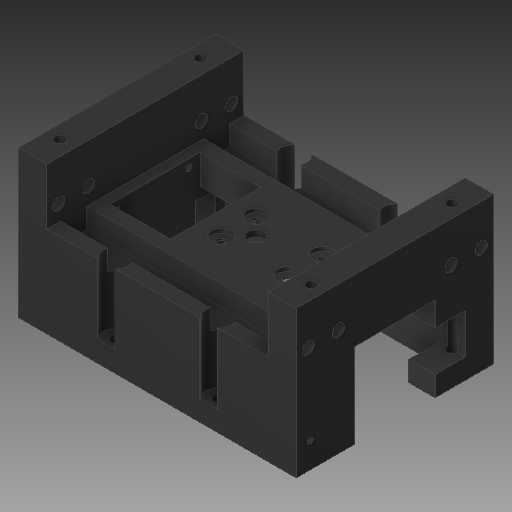
# Autodesk Inventor part: GA01
Saved by Autodesk Inventor 2017 (Build 210142000, 142)
## iProperties
Created: 2018-10-23
Part Number: GA01
Material: ABS Plastic
Document SubType Name: Modeling
Designer: Dell
Density: 1.06 g/cm^3
Appearance: Smooth - Black
Author: Dell
Autodesk Inventor part; units mm, degrees
ref_plane "YZ Plane" through (0, 0, 0) normal (1, 0, 0) x (0, 1, 0)
ref_plane "XZ Plane" through (0, 0, 0) normal (0, 1, 0) x (-1, 0, 0)
sketch "Sketch26" plane through (0, 0, 0) normal (0, 0, 1) x (1, 0, 0)
  line L0 (0, 0) -> (140, 0)
  line L1 (140, 0) -> (140, 48)
  line L2 (140, 48) -> (0, 48)
  line L3 (0, 48) -> (0, 0)
  dimension "d137" = 48
  dimension "d138" = 140
  constraints: 8 end point, 2 parallel, 1 horizontal, 1 perpendicular
  measures "d137" distance of L1.end L0.end
  measures "d138" distance of L1.end L2.end
extrude "Extrusion22" add sketch "Sketch26" along normal blind 100
sketch "Sketch27" plane through (0, 48, 0) normal (0, 1, 0) x (1, 0, 0)
  line L0 (0, -100) -> (140, -100) projected
  line L1 (0, 0) -> (140, 0) projected
  line L2 (15, -100) -> (125, -100)
  line L3 (125, -100) -> (125, 0)
  line L4 (125, 0) -> (15, 0)
  line L5 (15, 0) -> (15, -100)
  line L6 (0, 0) -> (0, -100) projected
  line L7 (140, -100) -> (0, -100) projected
  point P0 (70, -100)
  point P1 (70, -100)
  dimension "d141" = 15
  constraints: 8 end point, 4 midpoint, 2 parallel, 2 point on line, 1 horizontal, 1 perpendicular
  measures "d141" distance between parallel lines of L6 L5
extrude "Extrusion23" cut sketch "Sketch27" against normal blind 28 contours L5 L1 L3 L0
sketch "Sketch28" plane through (140, 0, 0) normal (1, 0, 0) x (0, 0, -1)
  circle A0 centre (-93, 28) radius 3
  circle A1 centre (-78, 28) radius 3
  line L0 (-93, 28) -> (-78, 28) construction
  line L1 (0, 48) -> (-100, 48) construction
  line L2 (-50, 48) -> (-50, 0) construction
  line L3 (0, 0) -> (-100, 0) construction
  line L4 (-100, 48) -> (0, 48) construction
  line L5 (-100, 20) -> (-100, 48) construction
  line L6 (-100, 20) -> (0, 20) construction
  line L7 (0, 48) -> (0, 20) construction
  circle A2 centre (-7, 28) radius 3
  circle A3 centre (-22, 28) radius 3
  dimension "d144" = 6
  dimension "d145" = 6
  dimension "d146" = 15
  dimension "d173" = 28
  dimension "d177" = 8
  constraints: 4 centre point, 4 end point, 2 midpoint, 2 symmetric about line, 1 horizontal, 2 other
  measures "d144" diameter of A0
  measures "d145" diameter of A1
  measures "d146" distance of L0.start L0.end
  measures "d173" distance from line of L2 L0.end
  measures "d177" distance from line of L6 L0.start
extrude "Extrusion24" cut sketch "Sketch28" against normal through all
sketch "Sketch30" plane through (0, 0, 0) normal (0, -1, 0) x (1, 0, 0)
  line L0 (63.5, 63.5) -> (39.5, 63.5) construction
  line L1 (39.5, 63.5) -> (39.5, 36.5) construction
  line L2 (39.5, 36.5) -> (63.5, 36.5) construction
  line L3 (63.5, 36.5) -> (63.5, 63.5) construction
  circle A0 centre (70, 50) radius 12.5
  line L4 (140, 0) -> (140, 100) projected
  line L5 (0, 100) -> (140, 100) projected
  circle A1 centre (63.5, 63.5) radius 1.5
  circle A2 centre (63.5, 36.5) radius 1.5
  circle A3 centre (55.5, 63.5) radius 1.5
  circle A4 centre (55.5, 36.5) radius 1.5
  circle A5 centre (47.5, 63.5) radius 1.5
  circle A6 centre (47.5, 36.5) radius 1.5
  circle A7 centre (39.5, 63.5) radius 1.5
  circle A8 centre (39.5, 36.5) radius 1.5
  point P0 (0, 0)
  point P1 (63.5, 50)
  point P2 (140, 50)
  point P3 (70, 100)
  dimension "d153" = 24
  dimension "d154" = 27
  dimension "d155" = 6.5
  dimension "d156" = 25
  dimension "d157" = 3
  dimension "d158" = 3
  dimension "d161" = 8
  constraints: 9 centre point, 8 end point, 3 midpoint, 2 coincident, 2 horizontal, 2 horizontal alignment, 2 parallel, 1 perpendicular, 1 vertical alignment, 12 other
  measures "d153" distance of L2.end L1.end
  measures "d154" distance of L1.end L0.end
  measures "d155" distance from line of L3 A0.centre
  measures "d156" diameter of A0
  measures "d157" diameter of A1
  measures "d158" diameter of A2
  measures "d161" distance of A1.centre A3.centre
extrude "Extrusion26" cut sketch "Sketch30" against normal through all
sketch "Sketch31" plane through (0, 0, 0) normal (0, -1, 0) x (1, 0, 0)
  line L0 (84, 70) -> (29, 70)
  line L1 (29, 70) -> (29, 30)
  line L2 (29, 30) -> (84, 30)
  line L3 (84, 30) -> (84, 70)
  circle A0 centre (70, 50) radius 12.5 projected
  point P0 (0, 0)
  point P1 (84, 50)
  dimension "d168" = 55
  dimension "d169" = 40
  dimension "d170" = 14
  constraints: 8 end point, 2 parallel, 1 horizontal, 1 horizontal alignment, 1 midpoint, 1 perpendicular
  measures "d168" distance of L1.end L2.end
  measures "d169" distance of L2.end L0.start
  measures "d170" distance from line of L3 A0.centre
extrude "Extrusion27" cut sketch "Sketch31" against normal blind 17 contours L3 L2 L1 L0 | A0
sketch "Sketch32" plane through (0, 0, 0) normal (0, -1, 0) x (1, 0, 0)
  line L0 (84, 30) -> (29, 30) projected
  line L1 (29, 30) -> (29, 70) projected
  line L2 (29, 70) -> (84, 70) projected
  line L3 (84, 70) -> (84, 30) projected
  line L4 (84, 30) -> (29, 30) projected
  line L5 (0, 0) -> (140, 0) projected
  line L6 (140, 0) -> (140, 100) projected
  line L7 (0, 100) -> (140, 100) projected
  line L8 (0, 0) -> (0, 100) projected
extrude "Extrusion28" add sketch "Sketch32" along normal blind 25
sketch "Sketch33" plane through (0, 20, 0) normal (0, 1, 0) x (1, 0, 0)
  circle A0 centre (70, -50) radius 12.5 construction
  line L0 (44.5, -94.1673) -> (19, -50) construction
  line L1 (19, -50) -> (44.5, -5.8327) construction
  line L2 (44.5, -5.8327) -> (95.5, -5.8327) construction
  line L3 (95.5, -5.8327) -> (121, -50) construction
  line L4 (121, -50) -> (95.5, -94.1673) construction
  line L5 (95.5, -94.1673) -> (44.5, -94.1673) construction
  circle A1 centre (121, -50) radius 2.5
  circle A2 centre (95.5, -94.1673) radius 2.5
  circle A3 centre (44.5, -94.1673) radius 2.5
  circle A4 centre (19, -50) radius 2.5
  circle A5 centre (44.5, -5.8327) radius 2.5
  circle A6 centre (95.5, -5.8327) radius 2.5
  point P0 (0, 0)
  point P1 (70, -50)
  dimension "d178" = 102
  dimension "d179" = 5
  dimension "d180" = 5
  dimension "d181" = 5
  dimension "d182" = 5
  dimension "d183" = 5
  dimension "d184" = 5
  constraints: 12 end point, 7 coincident, 6 centre point, 1 horizontal, 13 other
  measures "d178" distance of L0.end L3.end
  measures "d179" diameter of A1
  measures "d180" diameter of A2
  measures "d181" diameter of A3
  measures "d182" diameter of A4
  measures "d183" diameter of A5
  measures "d184" diameter of A6
extrude "Extrusion29" cut sketch "Sketch33" against normal through all
sketch "Sketch34" plane through (0, 20, 0) normal (0, 1, 0) x (1, 0, 0)
  circle A0 centre (70, -50) radius 12.5 projected
  circle A1 centre (95.5, -5.8327) radius 2.5 projected
  circle A2 centre (95.5, -5.8327) radius 6.5
  circle A3 centre (44.5, -5.8327) radius 6.5
  circle A4 centre (19, -50) radius 6.5
  circle A5 centre (44.5, -94.1673) radius 6.5
  circle A6 centre (95.5, -94.1673) radius 6.5
  circle A7 centre (121, -50) radius 6.5
  point P0 (0, 0)
  dimension "d187" = 13
  dimension "d190" = 360
  constraints: 6 centre point, 1 coincident, 13 other
  measures "d187" diameter of A2
extrude "Extrusion30" cut sketch "Sketch34" along normal blind 50 and the other way blind 35 contours A0 | A1 | A2 | A3 | A4 | A5 | A6 | A7
sketch "Sketch35" plane through (0, -25, 0) normal (0, -1, 0) x (1, 0, 0)
  circle A0 centre (44.5, 5.8327) radius 2.5 construction
  circle A1 centre (44.5, 94.1673) radius 2.5 construction
  circle A2 centre (121, 50) radius 2.5 construction
  circle A3 centre (95.5, 94.1673) radius 2.5 construction
  circle A4 centre (19, 50) radius 2.5 construction
  circle A5 centre (95.5, 5.8327) radius 2.5 construction
  line L0 (29, 70) -> (84, 70) projected
  line L1 (84, 70) -> (84, 30) projected
  line L2 (84, 30) -> (29, 30) projected
  line L3 (29, 30) -> (29, 70) projected
  line L4 (0, 0) -> (140, 0) construction
  line L5 (140, 0) -> (140, 100) construction
  line L6 (140, 100) -> (0, 100) construction
  line L7 (0, 100) -> (0, 0) construction
  line L8 (84, 30) -> (111, 30)
  line L9 (111, 30) -> (111, 70)
  line L10 (111, 70) -> (84, 70)
  line L11 (84, 70) -> (84, 30)
  dimension "d196" = 27
  constraints: 8 end point, 2 parallel, 1 horizontal, 1 horizontal alignment, 1 perpendicular
  measures "d196" distance of L1.end L8.end
extrude "Extrusion31" cut sketch "Sketch35" against normal blind 25 contours L10 L9 L8 L1
sketch "Sketch36" plane through (140, 48, 100) normal (0, 1, 0) x (1, 0, 0)
  line L0 (-7.5, 15) -> (-7.5, 85) construction
  circle A0 centre (-7.5, 15) radius 2.5
  circle A1 centre (-7.5, 85) radius 2.5
  line L1 (0, 0) -> (-15, 0) construction
  line L2 (0, 100) -> (0, 0) construction
  circle A2 centre (-70, 50) radius 12.5 construction
  line L3 (-70, 50) -> (-70, 0) construction
  line L4 (-47.3687, 0) -> (-92.6313, 0) construction
  circle A3 centre (-132.5, 15) radius 2.5
  circle A4 centre (-132.5, 85) radius 2.5
  point P0 (-7.5, 50)
  point P1 (-7.5, 0)
  point P2 (0, 50)
  dimension "d199" = 5
  dimension "d200" = 5
  dimension "d201" = 70
  constraints: 4 centre point, 4 end point, 4 midpoint, 2 coincident, 2 symmetric about line, 2 vertical, 1 horizontal alignment, 1 vertical alignment, 2 other
  measures "d199" diameter of A0
  measures "d200" diameter of A1
  measures "d201" distance of L0.start L0.end
extrude "Extrusion32" cut sketch "Sketch36" against normal through all
sketch "Sketch37" plane through (0, 0, 0) normal (0, -1, 0) x (1, 0, 0)
  line L0 (84, 62.0836) -> (140, 62.0836)
  line L1 (140, 62.0836) -> (140, 82.0836)
  line L2 (140, 82.0836) -> (84, 82.0836)
  line L3 (84, 82.0836) -> (84, 62.0836)
  arc A0 (92.6313, 100) -> (98.3687, 100) centre (95.5, 94.1673) ccw construction
  arc A1 (125, 55.1235) -> (125, 44.8765) centre (121, 50) ccw construction
  line L4 (95.5, 94.1673) -> (121, 94.1673) construction
  line L5 (121, 94.1673) -> (121, 50) construction
  line L6 (84, 70) -> (84, 30) projected
  line L7 (140, 0) -> (140, 100) projected
  point P0 (0, 0)
  point P1 (84, 72.0836)
  point P2 (121, 72.0836)
  dimension "d204" = 20
  constraints: 12 end point, 2 horizontal, 2 midpoint, 2 parallel, 2 perpendicular, 2 point on line, 1 horizontal alignment
  measures "d204" distance of L0.end L1.end
extrude "Extrusion33" cut sketch "Sketch37" along normal blind 20
sketch "Sketch38" plane through (0, 48, 100) normal (0, 1, 0) x (1, 0, 0)
  line L0 (15, 0) -> (0, 0) projected
  line L1 (140, 100) -> (125, 100) projected
  line L2 (0, 100) -> (0, 0) projected
  line L3 (140, 100) -> (140, 0) projected
  line L4 (0, 0) -> (140, 0)
  line L5 (140, 0) -> (140, 100)
  line L6 (140, 100) -> (0, 100)
  line L7 (0, 100) -> (0, 0)
  line L8 (139, 1) -> (1, 1)
  line L9 (1, 1) -> (1, 99)
  line L10 (1, 99) -> (139, 99)
  line L11 (139, 99) -> (139, 1)
  dimension "d207" = 1
  constraints: 16 end point, 4 parallel, 2 perpendicular, 1 horizontal, 3 other
  measures "d207" distance between parallel lines of L4 L8
extrude "Extrusion34" cut sketch "Sketch38" against normal through all
sketch "Sketch39" plane through (0, 0, 0) normal (0, -1, 0) x (1, 0, 0)
  line L0 (139, 62.0836) -> (139, 82.0836) projected
  line L1 (139, 82.0836) -> (84, 82.0836) projected
  line L2 (84, 82.0836) -> (84, 70) projected
  line L3 (84, 30) -> (84, 70) projected
  line L4 (111, 30) -> (84, 30) projected
  line L5 (111, 62.0836) -> (111, 30) projected
  line L6 (111, 62.0836) -> (139, 62.0836) projected
  arc A0 (48.8468, 1) -> (40.1532, 1) centre (44.5, 5.8327) ccw projected
  arc A1 (99.8468, 1) -> (91.1532, 1) centre (95.5, 5.8327) ccw projected
  arc A2 (40.1532, 99) -> (48.8468, 99) centre (44.5, 94.1673) ccw projected
  circle A3 centre (19, 50) radius 6.5 projected
  arc A4 (91.1532, 99) -> (99.8468, 99) centre (95.5, 94.1673) ccw projected
  circle A5 centre (121, 50) radius 6.5 projected
  line L7 (127.5, 82.0836) -> (19, 82.0836)
  line L8 (19, 82.0836) -> (19, 86.1673)
  line L9 (19, 86.1673) -> (127.5, 86.1673)
  line L10 (127.5, 86.1673) -> (127.5, 82.0836)
  line L11 (29, 70) -> (84, 70) projected
  line L12 (84, 70) -> (19, 70)
  line L13 (19, 70) -> (19, 82.0836)
  line L14 (19, 82.0836) -> (84, 82.0836)
  line L15 (84, 82.0836) -> (84, 70)
  line L16 (111, 42) -> (127.5, 42)
  line L17 (127.5, 42) -> (127.5, 13.8327)
  line L18 (127.5, 13.8327) -> (111, 13.8327)
  line L19 (111, 13.8327) -> (111, 42)
  line L20 (127.5, 13.8327) -> (19, 13.8327)
  line L21 (19, 13.8327) -> (19, 30)
  line L22 (19, 30) -> (127.5, 30)
  line L23 (127.5, 30) -> (127.5, 13.8327)
  circle A6 centre (132.5, 85) radius 2.5 projected
  point P0 (0, 0)
  point P1 (29, 30)
  dimension "d210" = 5
  dimension "d211" = 8
  dimension "d212" = 8
  dimension "d213" = 8
  constraints: 32 end point, 8 parallel, 4 horizontal, 4 perpendicular, 3 point on line, 3 vertical alignment
  measures "d210" distance from line of L10 A6.centre
  measures "d211" distance from line of A0.centre L20
  measures "d212" distance from line of L16 A5.centre
  measures "d213" distance from line of A2.centre L9
extrude "Extrusion35" cut sketch "Sketch39" along normal through all contours L6 L5 L4 L3 L2 L1 L0 | L1 L7 L8 L9 L10 | L2 L11 L12 L13 L7 | L19 L20 L21 L22 L4 | L22 L17 L18 L19
sketch "Sketch41" plane through (1, 48, 1) normal (-1, 0, 0) x (0, 0, 1)
  line L0 (69, -48) -> (69, -73) projected
  line L1 (69, -48) -> (69, -73) projected
  line L2 (29, -73) -> (29, -48) projected
  line L3 (29, -48) -> (29, -73) projected
  line L4 (29, -73) -> (29, -48) projected
  line L5 (29, -48) -> (69, -48)
  line L6 (69, -48) -> (69, -73)
  line L7 (69, -73) -> (29, -73)
  line L8 (29, -73) -> (29, -48)
  line L9 (29, -48) -> (19, -48)
  line L10 (19, -48) -> (19, -73)
  line L11 (19, -73) -> (29, -73)
  line L12 (29, -73) -> (29, -48)
  point P0 (-1, -48)
  dimension "d218" = 10
  constraints: 16 end point, 4 parallel, 2 horizontal, 2 perpendicular, 1 horizontal alignment
  measures "d218" distance between parallel lines of L10 L2
extrude "Extrusion36" cut sketch "Sketch41" against normal blind 5 contours L0 L7 L2 L5
extrude "Extrusion37" cut sketch "Sketch41" against normal blind 20 contours L2 L11 L10 L9
sketch "Sketch42" plane through (0, 0, 0) normal (0, -1, 0) x (1, 0, 0)
  line L0 (29, 70) -> (84, 70) projected
  line L1 (19, 86.1673) -> (19, 70) projected
  line L2 (29, 70) -> (19, 70)
  line L3 (19, 70) -> (19, 86.1673)
  line L4 (19, 86.1673) -> (29, 86.1673)
  line L5 (29, 86.1673) -> (29, 70)
  point P0 (0, 0)
  constraints: 8 end point, 2 parallel, 1 horizontal, 1 perpendicular
extrude "Extrusion38" add sketch "Sketch42" along normal blind 25
sketch "Sketch43" plane through (0, 0, 0) normal (0, -1, 0) x (1, 0, 0)
  line L0 (111, 62.0836) -> (111, 30) projected
  line L1 (127.5, 13.8327) -> (19, 13.8327) projected
  line L2 (111, 30) -> (127.5, 30)
  line L3 (127.5, 30) -> (127.5, 13.8327)
  line L4 (127.5, 13.8327) -> (111, 13.8327)
  line L5 (111, 13.8327) -> (111, 30)
  point P0 (0, 0)
  constraints: 8 end point, 2 parallel, 1 horizontal, 1 perpendicular
extrude "Extrusion39" add sketch "Sketch43" along normal blind 25
sketch "Sketch44" plane through (0, 0, 0) normal (0, -1, 0) x (1, 0, 0)
  line L0 (139, 62.0836) -> (111, 62.0836) projected
  line L1 (111, 62.0836) -> (111, 13.8327) projected
  line L2 (139, 62.0836) -> (111, 62.0836)
  line L3 (111, 62.0836) -> (111, 57.0836)
  line L4 (111, 57.0836) -> (139, 57.0836)
  line L5 (139, 57.0836) -> (139, 62.0836)
  point P0 (0, 0)
  dimension "d225" = 5
  constraints: 8 end point, 2 parallel, 1 horizontal, 1 perpendicular, 1 point on line
  measures "d225" distance between parallel lines of L4 L0
extrude "Extrusion40" cut sketch "Sketch44" along normal through all
sketch "Sketch45" plane through (0, 0, 0) normal (0, -1, 0) x (1, 0, 0)
  line L0 (127.5, 82.0836) -> (139, 82.0836) projected
  line L1 (139, 82.0836) -> (139, 57.0836) projected
  line L2 (127.5, 82.0836) -> (139, 82.0836)
  line L3 (139, 82.0836) -> (139, 77.0836)
  line L4 (139, 77.0836) -> (127.5, 77.0836)
  line L5 (127.5, 77.0836) -> (127.5, 82.0836)
  point P0 (0, 0)
  dimension "d228" = 5
  constraints: 8 end point, 2 parallel, 1 horizontal, 1 perpendicular, 1 point on line
  measures "d228" distance between parallel lines of L0 L4
extrude "Extrusion41" add sketch "Sketch45" along normal blind 25
sketch "Sketch46" plane through (0, 0, 0) normal (0, -1, 0) x (1, 0, 0)
  line L0 (127.5, 77.0836) -> (139, 77.0836) projected
  line L1 (29, 86.1673) -> (127.5, 86.1673) projected
  line L2 (127.5, 77.0836) -> (29, 77.0836)
  line L3 (29, 77.0836) -> (29, 86.1673)
  line L4 (29, 86.1673) -> (127.5, 86.1673)
  line L5 (127.5, 86.1673) -> (127.5, 77.0836)
  point P0 (0, 0)
  constraints: 8 end point, 2 parallel, 1 horizontal, 1 perpendicular
extrude "Extrusion42" add sketch "Sketch46" along normal blind 25
sketch "Sketch47" plane through (0, 0, 0) normal (0, -1, 0) x (1, 0, 0)
  line L0 (29, 30) -> (29, 70) projected
  line L1 (29, 77.0836) -> (139, 77.0836) projected
  line L2 (29, 70) -> (84, 70)
  line L3 (84, 70) -> (84, 77.0836)
  line L4 (84, 77.0836) -> (29, 77.0836)
  line L5 (29, 77.0836) -> (29, 70)
  point P0 (0, 0)
  constraints: 8 end point, 2 parallel, 1 horizontal, 1 midpoint, 1 perpendicular
extrude "Extrusion43" add sketch "Sketch47" along normal blind 25
sketch "Sketch48" plane through (0, 0, 0) normal (0, -1, 0) x (1, 0, 0)
  line L0 (84, 77.0836) -> (84, 70) construction
  line L1 (84, 30) -> (84, 70) construction
  line L2 (29, 30) -> (84, 30) construction
  line L3 (29, 30) -> (6, 30) construction
  line L4 (6, 30) -> (6, 70) construction
  line L5 (1, 70) -> (6, 70) construction
  line L6 (1, 20) -> (1, 70) construction
  line L7 (1, 20) -> (19, 20) construction
  line L8 (19, 20) -> (19, 13.8327) construction
  line L9 (19, 13.8327) -> (111, 13.8327) construction
  line L10 (111, 13.8327) -> (111, 57.0836) construction
  line L11 (111, 57.0836) -> (139, 57.0836) construction
  line L12 (139, 77.0836) -> (139, 57.0836) construction
  line L13 (139, 77.0836) -> (84, 77.0836) construction
  circle A0 centre (97.5, 25.4582) radius 1.5
  circle A1 centre (97.5, 40.4582) radius 1.5
  line L14 (111, 57.0836) -> (84, 57.0836) construction
  line L15 (84, 70) -> (84, 30) construction
  line L16 (97.5, 25.4582) -> (97.5, 40.4582) construction
  point P0 (0, 0)
  point P1 (97.5, 57.0836)
  point P2 (97.5, 32.9582)
  point P3 (111, 35.4582)
  dimension "d235" = 3
  dimension "d236" = 3
  dimension "d276" = 11.6255
  dimension "d277" = 15
  constraints: 4 end point, 3 midpoint, 2 centre point, 1 perpendicular, 1 point on line, 1 vertical, 1 vertical alignment
  measures "d235" diameter of A0
  measures "d236" diameter of A1
  measures "d276" distance from line of L9 L16.start
  measures "d277" distance of L16.start L16.end
extrude "Extrusion44" cut sketch "Sketch48" against normal blind 12
sketch "Sketch49" plane through (6, 48, 1) normal (-1, 0, 0) x (0, 0, 1)
  line L0 (69, -48) -> (69, -73) projected
  line L1 (29, -48) -> (69, -48) projected
  line L2 (29, -73) -> (29, -48) projected
  line L3 (69, -73) -> (29, -73) projected
  circle A0 centre (34, -68) radius 1.5
  circle A1 centre (64, -68) radius 1.5
  point P0 (-1, -48)
  dimension "d240" = 3
  dimension "d241" = 3
  dimension "d244" = 5
  dimension "d245" = 5
  dimension "d260" = 5
  constraints: 2 centre point, 1 horizontal alignment
  measures "d240" diameter of A0
  measures "d241" diameter of A1
  measures "d244" distance from line of L0 A1.centre
  measures "d245" distance from line of L3 A1.centre
  measures "d260" distance from line of L2 A0.centre
extrude "Extrusion45" cut sketch "Sketch49" against normal blind 25 contours A0 | A1
sketch "Sketch50" plane through (1, 48, 1) normal (-1, 0, 0) x (0, 0, 1)
  circle A0 centre (91, -60.5) radius 1.5
  circle A1 centre (7, -60.5) radius 1.5
  line L0 (69, -48) -> (69, -73) projected
  line L1 (0, 0) -> (0, -73) projected
  line L2 (98, 0) -> (98, -73) projected
  point P0 (-1, -48)
  point P1 (69, -60.5)
  point P2 (69, -60.5)
  dimension "d248" = 3
  dimension "d249" = 3
  dimension "d250" = 7
  dimension "d251" = 7
  constraints: 2 centre point, 2 horizontal alignment, 2 midpoint
  measures "d248" diameter of A0
  measures "d249" diameter of A1
  measures "d250" distance from line of L1 A1.centre
  measures "d251" distance from line of L2 A0.centre
extrude "Extrusion46" cut sketch "Sketch50" against normal blind 12
sketch "Sketch52" plane through (0, 0, 0) normal (0, -1, 0) x (1, 0, 0)
  circle A0 centre (97.5, 25.4582) radius 1.5 projected
  circle A1 centre (97.5, 40.4582) radius 1.5 projected
  line L0 (84, 77.0836) -> (84, 70) projected
  line L1 (84, 30) -> (84, 70) projected
  line L2 (29, 30) -> (84, 30) projected
  line L3 (29, 30) -> (6, 30) projected
  line L4 (6, 30) -> (6, 70) projected
  line L5 (1, 70) -> (6, 70) projected
  line L6 (1, 20) -> (1, 70) projected
  line L7 (1, 20) -> (19, 20) projected
  line L8 (19, 20) -> (19, 13.8327) projected
  line L9 (19, 13.8327) -> (111, 13.8327) projected
  line L10 (111, 13.8327) -> (111, 57.0836) projected
  line L11 (111, 57.0836) -> (139, 57.0836) projected
  line L12 (139, 77.0836) -> (139, 57.0836) projected
  line L13 (139, 77.0836) -> (84, 77.0836) projected
  line L14 (138, 58.0836) -> (85, 58.0836)
  line L15 (85, 58.0836) -> (85, 76.0836)
  line L16 (85, 76.0836) -> (138, 76.0836)
  line L17 (138, 76.0836) -> (138, 58.0836)
  line L18 (85, 76.0836) -> (110, 76.0836)
  line L19 (110, 76.0836) -> (110, 15.0836)
  line L20 (110, 15.0836) -> (85, 15.0836)
  line L21 (85, 15.0836) -> (85, 76.0836)
  point P0 (0, 0)
  dimension "d254" = 18
  dimension "d255" = 53
  dimension "d256" = 43
  dimension "d257" = 25
  dimension "d258" = 1
  dimension "d259" = 1
  constraints: 16 end point, 4 parallel, 2 horizontal, 2 perpendicular
  measures "d254" distance of L16.end L14.start
  measures "d255" distance of L15.end L16.end
  measures "d256" distance between parallel lines of L14 L20
  measures "d257" distance of L19.end L20.end
  measures "d258" distance from line of L0.end L21
  measures "d259" distance between parallel lines of L13 L16
sketch "Sketch54" plane through (0, 17, 0) normal (0, -1, 0) x (1, 0, 0)
  circle A0 centre (70, 50) radius 12.5 construction
  line L0 (36.7, 60) -> (61.2, 60) construction
  line L1 (61.2, 60) -> (61.2, 40)
  line L2 (61.2, 40) -> (36.7, 40)
  line L3 (36.7, 40) -> (36.7, 60)
  line L4 (62.2, 61) -> (35.7, 61)
  line L5 (35.7, 61) -> (35.7, 39)
  line L6 (35.7, 39) -> (62.2, 39)
  line L7 (62.2, 39) -> (62.2, 61)
  point P0 (61.2, 50)
  dimension "d278" = 8.8
  dimension "d279" = 20
  dimension "d280" = 24.5
  dimension "d281" = 1
  constraints: 16 end point, 4 parallel, 2 perpendicular, 1 horizontal, 1 horizontal alignment, 1 midpoint, 3 other
  measures "d278" distance from line of A0.centre L1
  measures "d279" distance of L2.end L0.start
  measures "d280" distance of L0.start L0.end
  measures "d281" distance between parallel lines of L0 L4
extrude "Extrusion47" cut sketch "Sketch54" against normal through all
sketch "Sketch55" plane through (0, 20, 0) normal (0, 1, 0) x (1, 0, 0)
  circle A0 centre (39.5, -36.5) radius 1.5 projected
  circle A1 centre (47.5, -36.5) radius 1.5 projected
  circle A2 centre (55.5, -36.5) radius 1.5 projected
  circle A3 centre (63.5, -36.5) radius 1.5 projected
  circle A4 centre (63.5, -63.5) radius 1.5 projected
  circle A5 centre (55.5, -63.5) radius 1.5 projected
  circle A6 centre (47.5, -63.5) radius 1.5 projected
  circle A7 centre (39.5, -63.5) radius 1.5 projected
  circle A8 centre (39.5, -36.5) radius 1.5 projected
  circle A9 centre (39.5, -36.5) radius 2.5
  circle A10 centre (47.5, -36.5) radius 1.5 projected
  circle A11 centre (47.5, -36.5) radius 2.5
  circle A12 centre (55.5, -36.5) radius 2.5
  circle A13 centre (63.5, -36.5) radius 2.5
  circle A14 centre (63.5, -63.5) radius 2.5
  circle A15 centre (55.5, -63.5) radius 1.5 projected
  circle A16 centre (55.5, -63.5) radius 2.5
  circle A17 centre (47.5, -63.5) radius 1.5 projected
  circle A18 centre (47.5, -63.5) radius 2.5
  circle A19 centre (39.5, -63.5) radius 2.5
  point P0 (0, 0)
  dimension "d284" = 5
  dimension "d285" = 5
  dimension "d286" = 5
  dimension "d287" = 5
  dimension "d288" = 5
  dimension "d289" = 5
  dimension "d290" = 5
  dimension "d291" = 5
  constraints: 8 centre point, 8 coincident
  measures "d284" diameter of A9
  measures "d285" diameter of A11
  measures "d286" diameter of A12
  measures "d287" diameter of A13
  measures "d288" diameter of A19
  measures "d289" diameter of A18
  measures "d290" diameter of A16
  measures "d291" diameter of A14
extrude "Extrusion48" cut sketch "Sketch55" against normal blind 2 contours A0 | A1 | A2 | A3 | A4 | A5 | A6 | A7 | A9 | A11 | A12 | A13 | A14 | A16 | A18 | A19
fillet "Fillet3" radius 2 2 edges at (62.2, 18.5, 59.7678) (62.2, 18.5, 40.2322)
sketch "Sketch56" plane through (0, 20, 0) normal (0, 1, 0) x (1, 0, 0)
  line L0 (1, -4) -> (1, -10)
  line L1 (15, -4) -> (15, -10)
  line L2 (1, -19) -> (1, -25)
  line L3 (15, -19) -> (15, -25)
  line L4 (125, -10) -> (125, -4)
  line L5 (15, -75) -> (15, -81)
  line L6 (15, -90) -> (15, -96)
  line L7 (15, -81) -> (15, -90)
  line L8 (15, -85.5) -> (125, -85.5)
  line L9 (15, -10) -> (15, -19)
  line L10 (15, -14.5) -> (125, -14.5)
  line L11 (15, -8) -> (125, -8)
  line L12 (125, -8) -> (125, -21)
  line L13 (125, -21) -> (15, -21)
  line L14 (15, -21) -> (15, -8)
  line L15 (15, -79) -> (125, -79)
  line L16 (125, -79) -> (125, -92)
  line L17 (125, -92) -> (15, -92)
  line L18 (15, -92) -> (15, -79)
  point P0 (0, 0)
  dimension "d295" = 13
  dimension "d296" = 13
  constraints: 38 end point, 6 midpoint, 4 parallel, 4 perpendicular, 4 point on line, 3 horizontal, 1 vertical
  measures "d295" distance between parallel lines of L13 L11
  measures "d296" distance between parallel lines of L17 L15
extrude "Extrusion49" cut sketch "Sketch56" against normal blind 10
sketch "Sketch57" plane through (0, 17, 0) normal (0, -1, 0) x (1, 0, 0)
  line L0 (29, 70) -> (84, 70) projected
  line L1 (84, 70) -> (139, 70)
  line L2 (139, 70) -> (139, 30)
  line L3 (139, 30) -> (84, 30)
  line L4 (84, 30) -> (84, 70)
  line L5 (29, 30) -> (84, 30) projected
  point P0 (0, 0)
  dimension "d299" = 55
  constraints: 8 end point, 3 point on line, 2 parallel, 1 horizontal, 1 perpendicular
  measures "d299" distance between parallel lines of L4 L2
extrude "Extrusion50" cut sketch "Sketch57" along normal through all
sketch "Sketch58" plane through (0, 17, 0) normal (0, -1, 0) x (1, 0, 0)
  arc A0 (64.0787, 38.9914) -> (64.0787, 61.0086) centre (70, 50) ccw projected
  line L0 (35.7, 61) -> (62.2, 61) projected
  circle A1 centre (121, 50) radius 6.5 projected
  arc A2 (62.2, 61) -> (64.0787, 61.0086) centre (63.1313, 62.7699) ccw projected
  arc A3 (64.0787, 38.9914) -> (64.0787, 61.0086) centre (70, 50) ccw projected
  arc A4 (64.0787, 38.9914) -> (62.2, 39) centre (63.1313, 37.2301) ccw projected
  line L1 (62.2, 39) -> (35.7, 39) projected
  line L2 (35.7, 39) -> (35.7, 61) projected
  line L3 (35.7, 61) -> (62.2, 61) projected
  line L4 (139, 70) -> (29, 70) construction
  line L5 (29, 30) -> (29, 70) projected
  line L6 (139, 30) -> (29, 30) projected
  circle A5 centre (39.5, 63.5) radius 1.5 projected
  circle A6 centre (47.5, 63.5) radius 1.5 projected
  circle A7 centre (55.5, 63.5) radius 1.5 projected
  circle A8 centre (63.5, 63.5) radius 1.5 projected
  circle A9 centre (63.5, 36.5) radius 1.5 projected
  circle A10 centre (55.5, 36.5) radius 1.5 projected
  circle A11 centre (47.5, 36.5) radius 1.5 projected
  circle A12 centre (39.5, 36.5) radius 1.5 projected
  circle A13 centre (70, 50) radius 4
  line L7 (139, 70) -> (139, 30) projected
  point P0 (0, 0)
  dimension "d302" = 8
  constraints: 1 centre point, 1 coincident
  measures "d302" diameter of A13
extrude "Extrusion51" add sketch "Sketch58" against normal blind 3 contours A4 L1 L2 L0 A2 A0 | A5 | A6 | A7 | A8 | A9 | A10 | A11 | A12
sketch "Sketch60" plane through (0, 20, 0) normal (0, 1, 0) x (1, 0, 0)
  arc A0 (64.8157, -38.6258) -> (64.3413, -38.8542) centre (63.5, -36.5) ccw projected
  circle A1 centre (55.5, -36.5) radius 2.5 projected
  circle A2 centre (47.5, -36.5) radius 1.5 projected
  circle A3 centre (47.5, -36.5) radius 2.5 projected
  circle A4 centre (39.5, -36.5) radius 2.5 projected
  circle A5 centre (39.5, -63.5) radius 2.5 projected
  circle A6 centre (47.5, -63.5) radius 2.5 projected
  circle A7 centre (55.5, -63.5) radius 2.5 projected
  arc A8 (64.3413, -61.1458) -> (64.8157, -61.3742) centre (63.5, -63.5) ccw projected
  arc A9 (64.8157, -38.6258) -> (64.3413, -38.8542) centre (70, -50) ccw projected
  arc A10 (64.8157, -38.6258) -> (64.3413, -38.8542) centre (63.5, -36.5) ccw projected
  circle A11 centre (63.5, -36.5) radius 1.5 projected
  arc A12 (64.3413, -61.1458) -> (64.8157, -61.3742) centre (70, -50) ccw projected
  arc A13 (64.3413, -61.1458) -> (64.8157, -61.3742) centre (63.5, -63.5) ccw projected
  circle A14 centre (63.5, -63.5) radius 1.5 projected
  point P0 (0, 0)
extrude "Extrusion52" add sketch "Sketch60" against normal blind 3 contours A9 A0 | A1 | A2 | A3 | A4 | A5 | A6 | A7 | A12 A8 | A11 | A14
sketch "Sketch61" plane through (0, 17, 0) normal (0, -1, 0) x (1, 0, 0)
  circle A0 centre (70, 50) radius 4 projected
  line L0 (94.5, 58.75) -> (61.5, 58.75) construction
  line L1 (61.5, 58.75) -> (61.5, 41.25) construction
  line L2 (61.5, 41.25) -> (94.5, 41.25) construction
  line L3 (94.5, 41.25) -> (94.5, 58.75) construction
  circle A1 centre (94.5, 58.75) radius 2
  circle A2 centre (61.5, 58.75) radius 2
  circle A3 centre (61.5, 41.25) radius 2
  circle A4 centre (94.5, 41.25) radius 2
  point P0 (0, 0)
  point P1 (94.5, 50)
  dimension "d307" = 33
  dimension "d308" = 17.5
  dimension "d309" = 8.5
  dimension "d310" = 4
  dimension "d311" = 4
  dimension "d312" = 4
  dimension "d313" = 4
  constraints: 8 end point, 4 centre point, 4 coincident, 2 parallel, 1 horizontal, 1 horizontal alignment, 1 midpoint, 1 perpendicular
  measures "d307" distance of L1.end L2.end
  measures "d308" distance of L2.end L0.start
  measures "d309" distance from line of L1 A0.centre
  measures "d310" diameter of A1
  measures "d311" diameter of A2
  measures "d312" diameter of A3
  measures "d313" diameter of A4
extrude "Extrusion53" cut sketch "Sketch61" against normal through all contours A1 | A2 | A3 | A4
sketch "Sketch62" plane through (0, 20, 0) normal (0, 1, 0) x (1, 0, 0)
  circle A0 centre (94.5, -41.25) radius 2 projected
  circle A1 centre (94.5, -58.75) radius 2 projected
  circle A2 centre (61.5, -58.75) radius 2 projected
  circle A3 centre (61.5, -41.25) radius 2 projected
  circle A4 centre (94.5, -41.25) radius 2 projected
  circle A5 centre (94.5, -41.25) radius 5
  circle A6 centre (94.5, -58.75) radius 5
  circle A7 centre (61.5, -41.25) radius 5
  circle A8 centre (61.5, -58.75) radius 2 projected
  circle A9 centre (61.5, -58.75) radius 5
  point P0 (0, 0)
  dimension "d316" = 10
  dimension "d317" = 10
  dimension "d318" = 10
  dimension "d319" = 10
  constraints: 4 centre point, 4 coincident
  measures "d316" diameter of A5
  measures "d317" diameter of A6
  measures "d318" diameter of A7
  measures "d319" diameter of A9
extrude "Extrusion54" cut sketch "Sketch62" against normal blind 2 contours A0 | A1 | A2 | A3 | A5 | A6 | A7 | A9
sketch "Sketch63" plane through (0, 0, 0) normal (0, -1, 0) x (1, 0, 0)
  line L0 (84, 70) -> (139, 70) projected
  line L1 (139, 77.0836) -> (139, 70) projected
  line L2 (139, 77.0836) -> (84, 77.0836) projected
  line L3 (84, 77.0836) -> (84, 70) projected
  line L4 (111, 30) -> (29, 30) projected
  line L5 (29, 30) -> (6, 30) projected
  line L6 (6, 30) -> (6, 70) projected
  line L7 (1, 70) -> (6, 70) projected
  line L8 (1, 20) -> (1, 70) projected
  line L9 (1, 20) -> (19, 20) projected
  line L10 (19, 20) -> (19, 13.8327) projected
  line L11 (19, 13.8327) -> (111, 13.8327) projected
  line L12 (111, 13.8327) -> (111, 30) projected
  circle A0 centre (97.5, 25.4582) radius 1.5 projected
  point P0 (0, 0)
extrude "Extrusion55" add sketch "Sketch63" along normal blind 25 contours L3 L2 L1 L0
sketch "Sketch64" plane through (29, 17, 70) normal (1, 0, 0) x (0, 0, -1)
  circle A0 centre (35, -37) radius 1.5 projected
  circle A1 centre (5, -37) radius 1.5 projected
  line L0 (0, 0) -> (0, -42) projected
  line L1 (40, -42) -> (0, -42) projected
  line L2 (40, -42) -> (40, -17) projected
  line L3 (40, -17) -> (40, 0) projected
  line L4 (40, 0) -> (0, 0) projected
  point P0 (70, -17)
extrude "Extrusion56" add sketch "Sketch64" along normal blind 21
sketch "Sketch66" plane through (0, -25, 0) normal (0, -1, 0) x (1, 0, 0)
  line L0 (20, 72.5) -> (50, 72.5)
  line L1 (50, 72.5) -> (50, 27.5)
  line L2 (50, 27.5) -> (20, 27.5)
  line L3 (20, 27.5) -> (20, 72.5)
  line L4 (50, 70) -> (50, 30) projected
  point P0 (0, 0)
  point P1 (50, 50)
  dimension "d328" = 30
  dimension "d329" = 45
  constraints: 8 end point, 2 midpoint, 2 parallel, 1 horizontal, 1 perpendicular
  measures "d328" distance of L1.end L2.end
  measures "d329" distance of L0.end L1.end
extrude "Extrusion57" cut sketch "Sketch66" against normal blind 45
sketch "Sketch67" plane through (0, -15, 0) normal (0, 1, 0) x (1, 0, 0)
  line L0 (20, -47.7087) -> (20, -43.5774) projected
  arc A0 (20, -43.5774) -> (20, -56.4226) centre (19, -50) ccw projected
  line L1 (20, -56.4226) -> (20, -52.2913) projected
  arc A1 (20, -47.7087) -> (20, -52.2913) centre (19, -50) ccw projected
  arc A2 (20, -47.7087) -> (20, -52.2913) centre (19, -50) ccw projected
  line L2 (20, -52.2913) -> (20, -47.7087)
  point P0 (0, 0)
  constraints: 2 end point, 1 vertical
extrude "Extrusion58" add sketch "Sketch67" along normal blind 35
sketch "Sketch68" plane through (0, 20, 0) normal (0, 1, 0) x (1, 0, 0)
  arc A0 (15, -44.8765) -> (15, -55.1235) centre (19, -50) ccw projected
  line L0 (15, -79) -> (15, -55.1235) projected
  line L1 (15, -55.1235) -> (15, -44.8765)
  point P0 (0, 0)
  constraints: 2 end point, 1 collinear
extrude "Extrusion59" add sketch "Sketch68" along normal blind 28
sketch "Sketch69" plane through (0, 20, 0) normal (0, 1, 0) x (1, 0, 0)
  arc A0 (125, -44.8765) -> (125, -55.1235) centre (121, -50) ccw projected
  arc A1 (125, -55.1235) -> (125, -44.8765) centre (121, -50) ccw projected
  point P0 (0, 0)
extrude "Extrusion60" add sketch "Sketch69" against normal blind 3
sketch "Sketch70" plane through (0, 20, 0) normal (0, 1, 0) x (1, 0, 0)
  arc A0 (125, -55.1235) -> (125, -44.8765) centre (121, -50) ccw projected
  line L0 (125, -21) -> (125, -44.8765) projected
  line L1 (125, -55.1235) -> (125, -44.8765)
  point P0 (0, 0)
  constraints: 2 end point, 1 vertical
extrude "Extrusion61" add sketch "Sketch70" along normal blind 28
sketch "Sketch71" plane through (0, -15, 0) normal (0, -1, 0) x (1, 0, 0)
  arc A0 (20, 52.2913) -> (20, 47.7087) centre (19, 50) ccw projected
  line L0 (20, 52.2913) -> (20, 47.7087) projected
  point P0 (0, 0)
extrude "Extrusion62" add sketch "Sketch71" along normal blind 10
sketch "Sketch72" plane through (20, -25, 72.5) normal (1, 0, 0) x (0, 0, -1)
  line L0 (39.25, 41) -> (3.25, 41) construction
  line L1 (3.25, 41) -> (3.25, 5) construction
  line L2 (3.25, 5) -> (39.25, 5) construction
  line L3 (39.25, 5) -> (39.25, 41) construction
  circle A0 centre (37.5, 5) radius 1.5 construction
  circle A1 centre (7.5, 5) radius 1.5 construction
  line L4 (0, 45) -> (45, 45) construction
  line L5 (0, 0) -> (0, 45) construction
  line L6 (42.5, 0) -> (0, 0) construction
  line L7 (42.5, 25) -> (42.5, 0) construction
  line L8 (45, 25) -> (42.5, 25) construction
  line L9 (45, 25) -> (45, 45) construction
  circle A2 centre (39.25, 41) radius 1.5
  circle A3 centre (3.25, 41) radius 1.5
  circle A4 centre (3.25, 5) radius 1.5
  circle A5 centre (39.25, 5) radius 1.5
  point P0 (72.5, 25)
  point P1 (21.25, 5)
  point P2 (21.25, 0)
  dimension "d342" = 36
  dimension "d343" = 36
  dimension "d344" = 5
  dimension "d345" = 3
  dimension "d346" = 3
  dimension "d347" = 3
  dimension "d348" = 3
  constraints: 8 end point, 4 centre point, 4 coincident, 2 midpoint, 2 parallel, 1 horizontal, 1 perpendicular, 1 vertical alignment
  measures "d342" distance of L2.end L1.end
  measures "d343" distance of L1.end L0.end
  measures "d344" distance between parallel lines of L6 L2
  measures "d345" diameter of A2
  measures "d346" diameter of A3
  measures "d347" diameter of A4
  measures "d348" diameter of A5
extrude "Extrusion63" cut sketch "Sketch72" against normal through all contours A2 | A3 | A4
sketch "Sketch73" plane through (0, 0, 0) normal (0, -1, 0) x (1, 0, 0)
  circle A0 centre (97.5, 25.4582) radius 1.5 projected
  point P0 (0, 0)
extrude "Extrusion64" add sketch "Sketch73" against normal blind 12
sketch "Sketch74" plane through (0, 0, 0) normal (0, -1, 0) x (1, 0, 0)
  line L0 (19, 20) -> (1, 20) projected
  line L1 (111, 13.8327) -> (19, 13.8327) projected
  line L2 (19, 20) -> (111, 20)
  line L3 (111, 20) -> (111, 13.8327)
  line L4 (111, 13.8327) -> (19, 13.8327)
  line L5 (19, 13.8327) -> (19, 20)
  line L6 (50, 30) -> (50, 27.5) projected
  line L7 (50, 30) -> (111, 30)
  line L8 (111, 30) -> (111, 20)
  line L9 (111, 20) -> (50, 20)
  line L10 (50, 20) -> (50, 30)
  point P0 (0, 0)
  constraints: 16 end point, 4 parallel, 2 horizontal, 2 perpendicular
extrude "Extrusion65" add sketch "Sketch74" along normal blind 25
ref_plane "Work Plane3" through (0, 5, 0) normal (0, 1, 0) x (1, 0, 0)
sketch "Sketch77" plane through (0, 5, 0) normal (0, 1, 0) x (1, 0, 0)
  line L0 (139, -30) -> (50, -30) projected
  line L1 (20, -30) -> (139, -30)
  line L2 (139, -30) -> (139, -15)
  line L3 (139, -15) -> (20, -15)
  line L4 (20, -15) -> (20, -30)
  point P0 (0, 0)
  dimension "d360" = 119
  dimension "d361" = 15
  constraints: 8 end point, 2 parallel, 1 horizontal, 1 perpendicular, 1 point on line
  measures "d360" distance of L3.end L2.end
  measures "d361" distance of L0.start L2.end
extrude "Extrusion66" cut sketch "Sketch77" against normal blind 20
sketch "Sketch79" plane through (0, 5, 0) normal (0, -1, 0) x (1, 0, 0)
  line L0 (50, 30) -> (139, 30) projected
  line L1 (126, 30) -> (139, 30)
  line L2 (139, 30) -> (139, 15.5)
  line L3 (139, 15.5) -> (126, 15.5)
  line L4 (126, 15.5) -> (126, 30)
  arc A0 (135, 15) -> (130, 15) centre (132.5, 15) ccw projected
  line L5 (139, 15) -> (135, 15) projected
  line L6 (139, 30) -> (139, 15) projected
  line L7 (50, 30) -> (139, 30) projected
  line L8 (50, 27.5) -> (50, 30) projected
  line L9 (20, 27.5) -> (50, 27.5) projected
  line L10 (20, 15) -> (20, 27.5) projected
  line L11 (130, 15) -> (20, 15) projected
  line L12 (139, 1) -> (139, 30) projected
  line L13 (20, 15) -> (126, 15)
  line L14 (126, 15) -> (126, 30)
  line L15 (126, 30) -> (20, 30)
  line L16 (20, 30) -> (20, 15)
  point P0 (0, 0)
  dimension "d364" = 6.5
  constraints: 16 end point, 4 parallel, 2 horizontal, 2 perpendicular, 1 midpoint, 1 point on line
  measures "d364" distance from line of L4 A0.centre
extrude "Extrusion67" cut sketch "Sketch79" along normal through all contours L0 L4 L14 L11 L10 L9 L8 | L8 L9 L16 L15
sketch "Sketch83" plane through (139, 48, 99) normal (1, 0, 0) x (0, 0, -1)
  circle A0 centre (7, -60.5) radius 1.5 projected
  point P0 (99, -48)
extrude "Extrusion68" cut sketch "Sketch83" against normal blind 16
body "Solid2"
